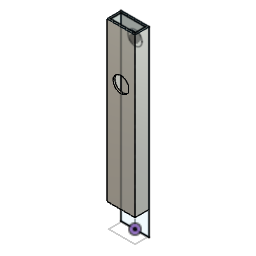
Intake+Support+arm (Autodesk Fusion 360 design; units mm, degrees)
Autodesk Fusion 360 part; units mm, degrees
sketch "Sketch1" plane through (0, 0, 0) normal (0, 0, 1) x (1, 0, 0)
  line L0 (0, 0) -> (0, 300.4312) construction
  circle A0 centre (0, 300.4312) radius 12.7
  line L1 (25.4, 0) -> (-25.4, 0)
  line L2 (-25.4, 0) -> (-25.4, 330.2)
  line L3 (-25.4, 330.2) -> (25.4, 330.2)
  line L4 (25.4, 330.2) -> (25.4, 0)
  dimension "d1" = 300.4312
  dimension "d2" = 25.4
  dimension "d3" = 50.8
  dimension "d4" = 330.2
  constraint coincident L0.start origin
  constraint vertical L0
  constraint coincident L0.end A0.centre
  constraint horizontal L1
  constraint vertical L2
  constraint horizontal L3
  constraint vertical L4
  constraint midpoint L0.start L1
  measures "d1" distance of L0.start L0.end
  measures "d2" diameter of A0
  measures "d3" distance of L1.start L1.end
  measures "d4" distance of L1.start L3.end
extrude "Extrude1" add sketch "Sketch1" along normal blind 25.4 contours A0 | L1 L2 L3 L4
sketch "Sketch2" plane through (0, 330.2, 0) normal (0, 1, 0) x (-1, 0, 0)
  line L0 (-25.4, 0) -> (25.4, 0)
  line L1 (25.4, 0) -> (25.4, 25.4)
  line L2 (25.4, 25.4) -> (-25.4, 25.4)
  line L3 (-25.4, 25.4) -> (-25.4, 0)
  line L4 (-22.225, 22.225) -> (-22.225, 3.175)
  line L5 (-22.225, 3.175) -> (22.225, 3.175)
  line L6 (22.225, 3.175) -> (22.225, 22.225)
  line L7 (22.225, 22.225) -> (-22.225, 22.225)
  dimension "d7" = -3.175
extrude "Extrude2" cut sketch "Sketch2" against normal up to surface (330.2 mm away) contours L4 L5 L6 L7
extrude "Extrude3" cut sketch "Sketch1" along normal blind 3.175 contours A0
move_face "OffsetFaces1" offset -43.4594 1 faces at (7.4083, 0, 1.0583)
sketch "Sketch3" plane through (0, 0, 0) normal (0, 0, 1) x (1, 0, 0)
  line L0 (-12.7, 300.4312) -> (-6.35, 289.4327) construction
  line L1 (-6.35, 289.4327) -> (6.35, 289.4327) construction
  line L2 (6.35, 289.4327) -> (12.7, 300.4312) construction
  line L3 (12.7, 300.4312) -> (6.35, 311.4297) construction
  line L4 (6.35, 311.4297) -> (-6.35, 311.4297) construction
  line L5 (-6.35, 311.4297) -> (-12.7, 300.4312) construction
  circle A0 centre (0, 300.4312) radius 30.48 construction
  circle A1 centre (0, 239.4712) radius 30.48 construction
  circle A2 centre (0, 239.4712) radius 14.2748
  point P0 (0, 300.4312)
  dimension "d19" = 12.7
  dimension "d20" = 60.96
  dimension "d21" = 60.96
  dimension "d22" = 28.5496
  constraint coincident P0 A0.centre
  constraint tangent A0 A1
  constraint concentric A1 A2
  measures "d19" distance of L0.start P0
  measures "d20" diameter of A0
  measures "d21" diameter of A1
  measures "d22" diameter of A2
extrude "Extrude5" cut sketch "Sketch3" along normal blind 50.8
component "Intake Support" placed x (1, 0, 0) y (0, 1, 0) z (0, 0, 1) at (0, 0, 0)
equation "d12 = -3 in + 1.289 in"
